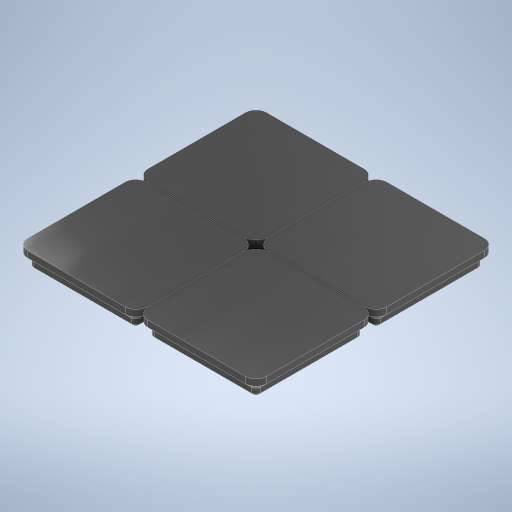
# Autodesk Inventor part: generic-module
Saved by Autodesk Inventor 2023 (Build 270158030, 158C)
## iProperties
Created: 2023-12-22
Part Number: generic-module
Material: Generic
Document SubType Name: Modeling
Designer: Imogen Heard
Density: 1 g/cm^3
Appearance: Dark Gray
Author: Imogen Heard
Autodesk Inventor part; units mm, degrees
ref_plane "YZ Plane" through (0, 0, 0) normal (1, 0, 0) x (0, 1, 0)
ref_plane "XZ Plane" through (0, 0, 0) normal (0, 1, 0) x (-1, 0, 0)
ref_plane "XY Plane" through (0, 0, 0) normal (0, 0, 1) x (1, 0, 0)
sketch "Sketch9" plane through (0, 0, 0) normal (0, 1, 0) x (-1, 0, 0)
  line L0 (-3.75, -41.5) -> (-37.75, -41.5)
  line L1 (-41.5, -37.75) -> (-41.5, -3.75)
  line L2 (-37.75, 0) -> (-3.75, 0)
  line L3 (0, -3.75) -> (0, -37.75)
  arc A0 (0, -3.75) -> (-3.75, 0) centre (-3.75, -3.75) ccw
  arc A1 (-37.75, 0) -> (-41.5, -3.75) centre (-37.75, -3.75) ccw
  arc A2 (-41.5, -37.75) -> (-37.75, -41.5) centre (-37.75, -37.75) ccw
  arc A3 (-3.75, -41.5) -> (0, -37.75) centre (-3.75, -37.75) ccw
  point P0 (0, 0)
  point P1 (0, -41.5)
  point P2 (-41.5, 0)
  point P3 (-41.5, -41.5)
  point P4 (0, 0)
  dimension "d50" = 41.5
  dimension "d51" = 41.5
  dimension "d52" = 3.75
  dimension "d55" = 3.75
  constraints: 8 end point, 8 point on circle, 8 point on line, 8 tangent, 4 centre point, 2 equal radius, 2 parallel, 1 coincident, 1 horizontal, 1 perpendicular
  measures "d50" distance between parallel lines of L1 L3
  measures "d51" distance between parallel lines of L2 L0
  measures "d52" radius of A0
  measures "d55" radius of A1
extrude "base-generic" add sketch "Sketch9" along normal blind 2.25
sketch "Sketch10" plane through (0, 0, 0) normal (0, -1, 0) x (1, 0, 0)
  line L0 (3.75, 0) -> (37.75, 0) projected
  arc A0 (3.75, 0) -> (0, -3.75) centre (3.75, -3.75) ccw projected
  line L1 (0, -37.75) -> (0, -3.75) projected
  arc A1 (0, -37.75) -> (3.75, -41.5) centre (3.75, -37.75) ccw projected
  line L2 (37.75, -41.5) -> (3.75, -41.5) projected
  arc A2 (37.75, -41.5) -> (41.5, -37.75) centre (37.75, -37.75) ccw projected
  line L3 (41.5, -3.75) -> (41.5, -37.75) projected
  arc A3 (41.5, -3.75) -> (37.75, 0) centre (37.75, -3.75) ccw projected
extrude "Extrusion8" add sketch "Sketch10" along normal blind 2.15 draft -45
sketch "Sketch11" plane through (0, -2.15, 0) normal (0, -1, 0) x (1, 0, 0)
  line L0 (37.75, -39.35) -> (3.75, -39.35) projected
  arc A0 (37.75, -39.35) -> (39.35, -37.75) centre (37.75, -37.75) ccw projected
  line L1 (39.35, -3.75) -> (39.35, -37.75) projected
  arc A1 (39.35, -3.75) -> (37.75, -2.15) centre (37.75, -3.75) ccw projected
  line L2 (3.75, -2.15) -> (37.75, -2.15) projected
  arc A2 (3.75, -2.15) -> (2.15, -3.75) centre (3.75, -3.75) ccw projected
  line L3 (2.15, -37.75) -> (2.15, -3.75) projected
  arc A3 (2.15, -37.75) -> (3.75, -39.35) centre (3.75, -37.75) ccw projected
  point P0 (0, 0)
extrude "Extrusion9" add sketch "Sketch11" along normal blind 1.8
sketch "Sketch12" plane through (0, -3.95, 0) normal (0, -1, 0) x (1, 0, 0)
  line L0 (37.75, -2.15) -> (3.75, -2.15) projected
  arc A0 (3.75, -2.15) -> (2.15, -3.75) centre (3.75, -3.75) ccw projected
  line L1 (2.15, -3.75) -> (2.15, -37.75) projected
  arc A1 (2.15, -37.75) -> (3.75, -39.35) centre (3.75, -37.75) ccw projected
  line L2 (3.75, -39.35) -> (37.75, -39.35) projected
  arc A2 (37.75, -39.35) -> (39.35, -37.75) centre (37.75, -37.75) ccw projected
  line L3 (39.35, -37.75) -> (39.35, -3.75) projected
  arc A3 (39.35, -3.75) -> (37.75, -2.15) centre (37.75, -3.75) ccw projected
  point P0 (0, 0)
extrude "Extrusion10" add sketch "Sketch12" along normal blind 0.8 draft -45
sketch "Sketch13" plane through (0, -4.75, 0) normal (0, -1, 0) x (1, 0, 0)
  circle A0 centre (7.75, -7.75) radius 3.25
  circle A1 centre (33.75, -7.75) radius 3.25
  circle A2 centre (33.75, -33.75) radius 3.25
  circle A3 centre (7.75, -33.75) radius 3.25
  line L0 (0, -37.75) -> (0, -3.75) projected
  line L1 (3.75, 0) -> (37.75, 0) projected
  line L2 (37.75, -41.5) -> (3.75, -41.5) projected
  line L3 (41.5, -3.75) -> (41.5, -37.75) projected
  point P0 (0, 0)
  dimension "d62" = 6.5
  dimension "d63" = 7.75
  dimension "d64" = 7.75
  dimension "d65" = 7.75
  dimension "d66" = 7.75
  constraints: 4 centre point, 3 equal radius, 2 horizontal alignment, 2 vertical alignment
  measures "d62" diameter of A0
  measures "d63" distance from line of L0 A0.centre
  measures "d64" distance from line of L1 A0.centre
  measures "d65" distance from line of L2 A3.centre
  measures "d66" distance from line of L3 A1.centre
extrude "Extrusion11" cut sketch "Sketch13" against normal blind 2.4
sketch "Sketch14" plane through (0, -4.75, 0) normal (0, -1, 0) x (1, 0, 0)
  circle A0 centre (7.75, -7.75) radius 1.5
  circle A1 centre (33.75, -7.75) radius 1.5
  circle A2 centre (33.75, -33.75) radius 1.5
  circle A3 centre (7.75, -33.75) radius 1.5
  circle A4 centre (7.75, -7.75) radius 3.25 projected
  circle A5 centre (33.75, -7.75) radius 3.25 projected
  circle A6 centre (33.75, -33.75) radius 3.25 projected
  circle A7 centre (7.75, -33.75) radius 3.25 projected
  point P0 (0, 0)
  dimension "d69" = 3
  constraints: 4 centre point, 4 concentric, 3 equal radius
  measures "d69" diameter of A0
extrude "Extrusion12" cut sketch "Sketch14" against normal blind 6 contours A0 | A1 | A2 | A3
pattern_linear "Rectangular Pattern1" count 2 spacing 42 along (0, 0, -1) count 2 spacing 42 along (-1, 0, 0)
equation "\"d51\" = d50"
equation "\"d64\" = d63"
equation "\"d65\" = d63"
equation "\"d66\" = d63"
body "Solid2"
